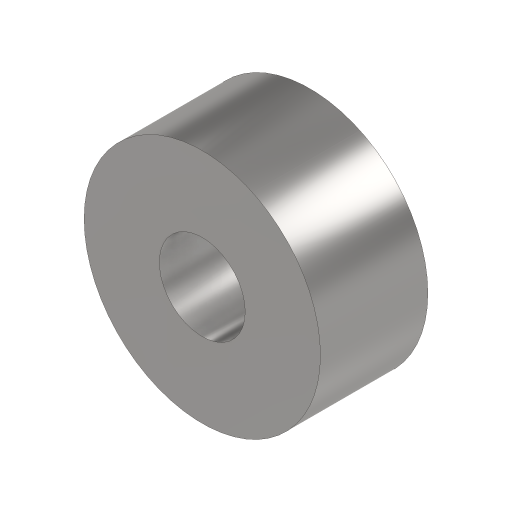
# Autodesk Inventor part: gear_pin_0824
Saved by Autodesk Inventor 2024 (Build 280153000, 153)
## iProperties
Created: 2022-10-17
Part Number: gear_pin_0824
Material: 不鏽鋼
Document SubType Name: Modeling
Designer: USER
Density: 8 g/cm^3
Appearance: 半拋光
Author: USER
Autodesk Inventor part; units mm, degrees
ref_plane "YZ Plane" through (0, 0, 0) normal (1, 0, 0) x (0, 1, 0)
ref_plane "XZ Plane" through (0, 0, 0) normal (0, 1, 0) x (-1, 0, 0)
ref_plane "XY Plane" through (0, 0, 0) normal (0, 0, 1) x (1, 0, 0)
sketch "草圖9" plane through (0, 0, 0) normal (0, 0, 1) x (1, 0, 0)
  circle A0 centre (0, 0) radius 4
  circle A1 centre (0, 0) radius 11
  dimension "d34" = 8
  dimension "d35" = 22
  constraints: 2 centre point, 2 coincident
  measures "d34" diameter of A0
  measures "d35" diameter of A1
extrude "擠出9" add sketch "草圖9" along normal blind 10
equation "\"模數\" = 0.9"
equation "\"PressureAngle\" = 20deg"
equation "\"UnitProfileClearance\" = 0.25"
equation "\"UnitRoundRadius\" = 0.35"
equation "\"HeadDiameter\" = 26.08158"
equation "\"RootDiameter\" = 22.05"
equation "\"BaseDiameter\" = 22.83453"
equation "\"PitchDiameter\" = 24.3"
equation "\"HelixAngle\" = 0"
equation "\"UnitCorrection\" = 0"
equation "\"UnitAddendumModification\" = 0.010235"
equation "\"CircularPitch\" = 2.82743"
equation "\"UnitBacklashShift\" = 0"
equation "\"TotalToolShift\" = 0"
equation "\"IsInternal\" = 0"
